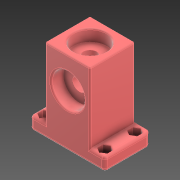
# Autodesk Inventor part: 3 dubbele lagerblok
Saved by Autodesk Inventor 2020 (Build 240168000, 168)
## iProperties
Created: 2020-05-19
Part Number: 3 dubbele lagerblok
Material: Generic
Document SubType Name: Modeling
Designer: stefa
Density: 1 g/cm^3
Appearance: Default
Author: stefa
Autodesk Inventor part; units mm, degrees
ref_plane "YZ Plane" through (0, 0, 0) normal (1, 0, 0) x (0, 1, 0)
ref_plane "XZ Plane" through (0, 0, 0) normal (0, 1, 0) x (-1, 0, 0)
ref_plane "XY Plane" through (0, 0, 0) normal (0, 0, 1) x (1, 0, 0)
sketch "Sketch1" plane through (0, 0, 0) normal (0, 1, 0) x (-1, 0, 0)
  line L0 (-15, 15) -> (15, 15)
  line L1 (15, 15) -> (15, -15)
  line L2 (15, -15) -> (-15, -15)
  line L3 (-15, -15) -> (-15, 15)
  line L4 (-15, 15) -> (15, -15) construction
  line L5 (15, 15) -> (-15, -15) construction
  circle A0 centre (11.5, 11.5) radius 1.5
  circle A1 centre (11.5, -11.5) radius 1.5
  circle A2 centre (-11.5, 11.5) radius 1.5
  circle A3 centre (-11.5, -11.5) radius 1.5
  point P0 (0, 0)
  dimension "d1" = 30
  dimension "d10" = 3
  dimension "d11" = 3.5
  dimension "d14" = 23
  dimension "d17" = 23
  dimension "d25" = 30
  constraints: 12 end point, 4 centre point, 2 horizontal, 2 midpoint, 2 parallel, 1 perpendicular, 1 point on line, 1 vertical, 6 other
  measures "d1" distance of L0.end L1.end
  measures "d10" diameter of A0
  measures "d11" distance from line of L1 A0.centre
  measures "d14" distance of A0.centre A1.centre
  measures "d17" distance of A0.centre A2.centre
  measures "d25" distance of L1.end L2.end
extrude "Extrusion1" add sketch "Sketch1" along normal mid plane 47 contours L0 L1 L2 L3 | A0 | A1 | A2 | A3
sketch "Sketch2" plane through (0, 23.5, 0) normal (0, 1, 0) x (1, 0, 0)
  circle A0 centre (0, 0) radius 11
  dimension "d4" = 22
  constraints: 1 centre point, 1 coincident
  measures "d4" diameter of A0
extrude "Extrusion2" cut sketch "Sketch2" against normal blind 8
sketch "Sketch3" plane through (-15, 23.5, 15) normal (0, 0, 1) x (1, 0, 0)
  circle A0 centre (15, -21) radius 11
  line L0 (0, 0) -> (30, 0) projected
  point P0 (15, -23.5)
  dimension "d7" = 22
  dimension "d27" = 21
  constraints: 1 centre point, 1 coincident, 1 vertical alignment
  measures "d7" diameter of A0
  measures "d27" distance from line of L0 point (15, -21)
extrude "Extrusion3" cut sketch "Sketch3" against normal blind 8
fillet "Fillet1" radius 1 2 edges at (-11, 23.5, 0) (-11, 2.5, 15)
fillet "Fillet2" radius 1 8 edges at (15, 0, 15) (15, 23.5, 0) (0, 23.5, 15) (15, 0, -15) (0, 23.5, -15) (-15, 0, -15) (-15, 23.5, 0) (-15, 0, 15)
sketch "Sketch5" plane through (0, -23.5, 0) normal (0, -1, 0) x (1, 0, 0)
  line L0 (-25, 15) -> (25, 15)
  line L1 (25, 15) -> (25, -15)
  line L2 (25, -15) -> (-25, -15)
  line L3 (-25, -15) -> (-25, 15)
  line L4 (-25, 15) -> (25, -15) construction
  line L5 (25, 15) -> (-25, -15) construction
  line L6 (23.325, 8.0803) -> (20, 6.1606)
  line L7 (20, 6.1606) -> (16.675, 8.0803)
  line L8 (16.675, 8.0803) -> (16.675, 11.9197)
  line L9 (16.675, 11.9197) -> (20, 13.8394)
  line L10 (20, 13.8394) -> (23.325, 11.9197)
  line L11 (23.325, 11.9197) -> (23.325, 8.0803)
  line L12 (-16.675, 8.0803) -> (-20, 6.1606)
  line L13 (-20, 6.1606) -> (-23.325, 8.0803)
  line L14 (-23.325, 8.0803) -> (-23.325, 11.9197)
  line L15 (-23.325, 11.9197) -> (-20, 13.8394)
  line L16 (-20, 13.8394) -> (-16.675, 11.9197)
  line L17 (-16.675, 11.9197) -> (-16.675, 8.0803)
  line L18 (23.325, -11.9197) -> (20, -13.8394)
  line L19 (20, -13.8394) -> (16.675, -11.9197)
  line L20 (16.675, -11.9197) -> (16.675, -8.0803)
  line L21 (16.675, -8.0803) -> (20, -6.1606)
  line L22 (20, -6.1606) -> (23.325, -8.0803)
  line L23 (23.325, -8.0803) -> (23.325, -11.9197)
  line L24 (-16.675, -11.9197) -> (-20, -13.8394)
  line L25 (-20, -13.8394) -> (-23.325, -11.9197)
  line L26 (-23.325, -11.9197) -> (-23.325, -8.0803)
  line L27 (-23.325, -8.0803) -> (-20, -6.1606)
  line L28 (-20, -6.1606) -> (-16.675, -8.0803)
  line L29 (-16.675, -8.0803) -> (-16.675, -11.9197)
  circle A0 centre (20, 10) radius 1.55
  circle A1 centre (-20, 10) radius 1.55
  circle A2 centre (20, -10) radius 1.55
  circle A3 centre (-20, -10) radius 1.55
  point P0 (0, 0)
  dimension "d28" = 50
  dimension "d29" = 30
  dimension "d53" = 6.65
  dimension "d54" = 5
  dimension "d55" = 5
  dimension "d58" = 40
  dimension "d61" = 20
  dimension "d67" = 3.1
  dimension "d70" = 40
  dimension "d73" = 20
  constraints: 60 end point, 4 centre point, 3 horizontal, 3 parallel, 2 coincident, 2 midpoint, 2 vertical, 1 perpendicular, 58 other
  measures "d28" distance of L1.end L2.end
  measures "d29" distance of L0.end L1.end
  measures "d53" distance between parallel lines of L11 L8
  measures "d54" distance from line of L0 point (20, 10)
  measures "d55" distance from line of L1 point (20, 10)
  measures "d58" distance of point (20, 10) point (-20, 10)
  measures "d61" distance of point (20, 10) point (20, -10)
  measures "d67" diameter of A0
  measures "d70" distance of A0.centre A1.centre
  measures "d73" distance of A0.centre A2.centre
extrude "Extrusion4" add sketch "Sketch5" along normal blind 9 contours L0 L1 L2 L3 | L6 L7 L8 L9 L10 L11 | L12 L13 L14 L15 L16 L17 | L18 L19 L20 L21 L22 L23 | L24 L25 L26 L27 L28 L29 | A0 | A1 | A2 | A3
fillet "Fillet3" radius 2 13 edges at (25, -28, -15) (-25, -28, -15) (-19.5, -23.5, -15) (-25, -23.5, 0) (25, -23.5, 0) (19.5, -23.5, 15) (-19.5, -23.5, 15) (0, -32.5, -15) (-25, -32.5, 0) (0, -32.5, 15) (25, -32.5, 0) (-25, -28, 15) (25, -28, 15)
sketch "Sketch6" plane through (0, 15.5, 0) normal (0, 1, 0) x (1, 0, 0)
  circle A0 centre (0, 0) radius 4.5
  dimension "d44" = 9
  constraints: 1 centre point, 1 coincident
  measures "d44" diameter of A0
extrude "Extrusion5" cut sketch "Sketch6" against normal blind 10
sketch "Sketch8" plane through (0, 2.5, 7) normal (0, 0, 1) x (1, 0, 0)
  circle A0 centre (0, 0) radius 11 projected
  circle A1 centre (0, 0) radius 4.5
  point P0 (0, -2.5)
  dimension "d50" = 9
  constraints: 1 centre point, 1 coincident
  measures "d50" diameter of A1
extrude "Extrusion7" cut sketch "Sketch8" against normal blind 10 contours A1
mirror "Mirror4" about plane through (0, 0, 0) normal (0, 0, 1) of "Extrusion3", "Extrusion7"
extrude "Extrusion8" cut sketch "Sketch5" along normal blind 4.5 contours L6 L7 L8 L9 L10 L11 | L12 L13 L14 L15 L16 L17 | L18 L19 L20 L21 L22 L23 | L24 L25 L26 L27 L28 L29 | A0 | A1 | A2 | A3
extrude "Extrusion9" cut sketch "Sketch5" along normal up to surface (9 mm away) contours A0 | A1 | A2 | A3
fillet "Fillet4" radius 0.2 38 edges at (-16.675, -23.5, -10) (-17.6106, -23.5, -12.4598) (-19.2905, -23.5467, -13.4297) (-22.2269, -23.5, -12.5537) (-23.163, -23.5067, -12.0132) (-20.7095, -23.5467, -13.4297) (-23.325, -23.5266, -10) (-23.163, -23.5067, -7.9868) (-21.5, -23.5, -7.0266) (-18.3375, -23.5, -7.1205) (-18.3375, -23.5, 7.1205) (-23.163, -23.5067, 7.9868) (-21.5, -23.5, 7.0266) (-23.325, -23.5266, 10) (-23.163, -23.5067, 12.0132) (-20.7095, -23.5467, 13.4297) (-22.2269, -23.5, 12.5537) (-17.6106, -23.5, 12.4598) (-19.2905, -23.5467, 13.4297) (-16.675, -23.5, 10) (23.163, -23.5067, 7.9868) (21.5, -23.5, 7.0266) (23.325, -23.5266, 10) (22.2269, -23.5, 12.5537) (23.163, -23.5067, 12.0132) (20.7095, -23.5467, 13.4297) (17.6106, -23.5, 12.4598) (19.2905, -23.5467, 13.4297) (16.675, -23.5, 10) (18.3375, -23.5, 7.1205) (18.3375, -23.5, -12.8795) (16.675, -23.5, -10) (23.163, -23.5067, -12.0132) (21.5, -23.5, -12.9734) (23.325, -23.5266, -10) (23.163, -23.5067, -7.9868) (21.5, -23.5, -7.0266) (18.3375, -23.5, -7.1205)
fillet "Fillet5" radius 0.3 4 edges at (-21.55, -32.5, 10) (-21.55, -32.5, -10) (18.45, -32.5, -10) (18.45, -32.5, 10)
equation "\"d14\" = d1 - 2 * d11"
equation "\"d17\" = d14"
equation "\"d58\" = d28 - 2 * d55"
equation "\"d61\" = d29 - 2 * d54"
equation "\"d70\" = d58"
equation "\"d73\" = d61"
body "Solid1"
